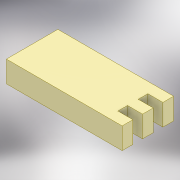
# Autodesk Inventor part: FVT LITTLEBEE BLHeli 20A ESC
Saved by Autodesk Inventor 2018 (Build 220112000, 112)
## iProperties
Created: 2018-01-09
Part Number: FVT LITTLEBEE BLHeli 20A ESC
Material: Nylon 6/6
Document SubType Name: Modeling
Designer: fbl92568
Density: 1.13 g/cm^3
Appearance: Nylon 6
Author: fbl92568
Autodesk Inventor part; units mm, degrees
ref_plane "YZ Plane" through (0, 0, 0) normal (1, 0, 0) x (0, 1, 0)
ref_plane "XZ Plane" through (0, 0, 0) normal (0, 1, 0) x (-1, 0, 0)
ref_plane "XY Plane" through (0, 0, 0) normal (0, 0, 1) x (1, 0, 0)
sketch "Sketch1" plane through (0, 0, 0) normal (0, 0, 1) x (1, 0, 0)
  line L0 (27, 12) -> (0, 12)
  line L1 (0, 12) -> (0, 0)
  line L2 (27, 12) -> (27, 9.5)
  line L3 (27, 9.5) -> (23.5, 9.5)
  line L4 (23.5, 2.5) -> (27, 2.5)
  line L5 (27, 2.5) -> (27, 0)
  line L6 (27, 0) -> (23.5, 0)
  line L7 (23.5, 7.25) -> (27, 7.25)
  line L8 (27, 7.25) -> (27, 4.75)
  line L9 (27, 4.75) -> (23.5, 4.75)
  line L10 (23.5, 2.5) -> (23.5, 4.75)
  line L11 (23.5, 7.25) -> (23.5, 9.5)
  line L12 (0, 0) -> (27, 0)
  dimension "d2" = 2.5
  dimension "d4" = 2.5
  dimension "d8" = 2.5
  dimension "d9" = 2.25
  dimension "d10" = 7
  dimension "d11" = 27
  dimension "d12" = 12
  dimension "d13" = 3.5
  dimension "d14" = 3.5
  dimension "d15" = 3.5
  constraints: 26 end point, 5 parallel, 3 horizontal, 2 collinear, 2 perpendicular
  measures "d2" distance of L0.start L2.end
  measures "d4" distance of L4.end L5.end
  measures "d8" distance of L7.end L8.end
  measures "d9" distance between parallel lines of L3 L7
  measures "d10" distance from line of L4.end L3
  measures "d11" distance between parallel lines of L1 L2
  measures "d12" distance of L0.end L1.end
  measures "d13" distance of L2.end L3.end
  measures "d14" distance of L8.end L9.end
  measures "d15" distance from line of L6.end L2
extrude "Extrusion1" add sketch "Sketch1" along normal blind 5
equation "\"d4\" = d2"
equation "\"d8\" = d2"
equation "\"d9\" = -0.5 * d8 + 0.5 * d10"
equation "\"d14\" = d13"
body "Solid1"
